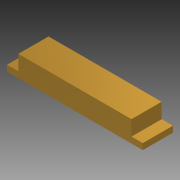
# Autodesk Inventor part: UNLHEP-14-01-P-012_StampPlate
Saved by Autodesk Inventor 2013 (Build 170138000, 138)
## iProperties
Created: 2014-01-23
Part Number: UNLHEP-14-01-P-012_StampPlate
Material: Messing, weicher Gelbton
Document SubType Name: Modeling
Designer: Frank Meier
Density: 8.47 g/cm^3
Mass: 174.482 g
Surface Area: 62.2 cm^2
Volume: 20.6 cm^3
Project: UNL Pixel Phase I
Author: Frank Meier
Autodesk Inventor part; units mm, degrees
ref_plane "YZ Plane" through (0, 0, 0) normal (1, 0, 0) x (0, 1, 0)
ref_plane "XZ Plane" through (0, 0, 0) normal (0, 1, 0) x (-1, 0, 0)
ref_plane "XY Plane" through (0, 0, 0) normal (0, 0, 1) x (1, 0, 0)
sketch "Skizze1" plane through (0, 0, 0) normal (0, 0, 1) x (1, 0, 0)
  line L0 (-45, -10) -> (45, -10)
  line L1 (45, -10) -> (45, 10)
  line L2 (45, 10) -> (-45, 10)
  line L3 (-45, 10) -> (-45, -10)
  line L4 (-45, -10) -> (45, 10) construction
  line L5 (45, -10) -> (-45, 10) construction
  point P0 (0, 0)
  dimension "d0" = 90
  dimension "d1" = 20
  constraints: 12 end point, 2 midpoint, 2 parallel, 1 horizontal, 1 perpendicular
  measures "d0" distance of L1.end L2.end
  measures "d1" distance of L0.end L1.end
extrude "Extrusion1" add sketch "Skizze1" along normal blind 4
sketch "Skizze2" plane through (0, 0, 4) normal (0, 0, 1) x (1, 0, 0)
  line L0 (45, 10) -> (-45, 10) projected
  line L1 (-37.5, -10) -> (37.5, -10)
  line L2 (37.5, -10) -> (37.5, 10)
  line L3 (37.5, 10) -> (-37.5, 10)
  line L4 (-37.5, 10) -> (-37.5, -10)
  line L5 (-37.5, -10) -> (37.5, 10) construction
  line L6 (37.5, -10) -> (-37.5, 10) construction
  point P0 (0, 0)
  dimension "d4" = 75
  constraints: 12 end point, 2 midpoint, 2 parallel, 1 horizontal, 1 perpendicular, 1 point on line
  measures "d4" distance of L2.end L3.end
extrude "Extrusion2" add sketch "Skizze2" along normal blind 10
